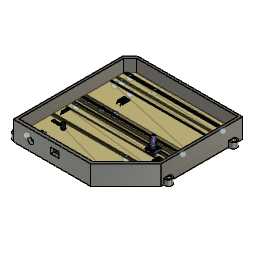
ECE198 Housing v1-4 (Autodesk Fusion 360 design; units mm, degrees)
Autodesk Fusion 360 part; units mm, degrees
note: some values were not read from the file. Set by a fixed rule: which sketch regions a step uses.
other "Base Mesh Feature1"
sketch "Sketch1" plane through (0, 0, 0) normal (0, 0, 1) x (1, 0, 0)
  line L0 (25, 15) -> (591.489777, 15)
  line L1 (401.489777, -615.270017) -> (-15, -615.270017)
  line L2 (591.489777, -425.270017) -> (401.489777, -615.270017)
  line L3 (25, 15) -> (-15, -25)
  line L4 (-15, -615.270017) -> (-15, -25)
  line L5 (-504.56746, -488.736197) -> (-504.56746, -504.009761)
  line L6 (-504.56746, -504.009761) -> (-694.56746, -694.009761)
  arc A0 (-1111.057237, -103.739744) -> (-1111.057237, -138.733703) centre (-1118.560257, -121.236724) ccw
  line L7 (-504.56746, -63.739744) -> (-504.56746, -103.73725)
  line L8 (-1071.057237, -63.739744) -> (-1111.057237, -103.739744)
  line L9 (-1111.057237, -653.739744) -> (-1111.057237, -688.733703)
  arc A1 (-504.573277, -138.733703) -> (-504.56746, -103.73725) centre (-497.070257, -121.236724) ccw
  line L10 (-504.56746, -453.73725) -> (-504.573277, -488.733703)
  arc A2 (-504.573277, -488.733703) -> (-504.56746, -453.73725) centre (-497.070257, -471.236724) ccw
  line L11 (-504.56746, -138.736197) -> (-504.56746, -453.73725)
  line L12 (-504.56746, -103.73725) -> (-504.56746, -138.736197)
  line L13 (-1111.057237, -653.739744) -> (-1111.057237, -138.733703)
  line L14 (-694.56746, -694.009761) -> (-1111.057237, -694.009761)
  arc A3 (-1111.057237, -653.739744) -> (-1111.057237, -688.733703) centre (-1118.560257, -671.236724) ccw
  line L15 (-1071.057237, -63.739744) -> (-504.56746, -63.739744)
  line L16 (-1111.057237, -138.733703) -> (-1111.057237, -103.739744)
  line L17 (-1111.057237, -694.009761) -> (-1111.057237, -688.733703)
  line L18 (591.489777, 15) -> (591.489777, -425.270017)
  point P0 (-15, 15)
  point P1 (591.489777, -615.270017)
  point P2 (-1111.057237, -63.739744)
  point P3 (-504.56746, -694.009761)
  point P4 (-1096.057237, -78.739744)
  dimension "d1" = 190
  dimension "d2" = 190
  dimension "d3" = 40
  dimension "d4" = 40
  dimension "d13" = 190
  dimension "d14" = 190
  dimension "d15" = 40
  dimension "d16" = 40
  constraint horizontal L0
  constraint horizontal L1
  constraint coincident P0 L0
  constraint horizontal L15
  constraint vertical L7
  constraint horizontal L14
  constraint vertical L17
  constraint collinear L13 L17
  constraint collinear L7 L11
  constraint collinear L5 L11
  constraint parallel L13 L16
  constraint perpendicular L0 L18
  measures "d3" distance of P0 L0.start
  measures "d4" distance of P0 L3.end
extrude "Extrude1" add sketch "Sketch1" against normal blind 30 contours L0 L1 L2 L3 L4 L18 picked at (402.659851, -131.756672) makes body 1
sketch "Sketch2" plane through (0, 0, 0) normal (0, 0, 1) x (-1, 0, 0)
  line L0 (-591.489777, -15) -> (-25, -15)
  line L1 (-25, -15) -> (15, 25)
  line L2 (15, 25) -> (15, 615.270017)
  line L3 (15, 615.270017) -> (-401.489777, 615.270017)
  line L4 (-401.489777, 615.270017) -> (-591.489777, 425.270017)
  line L5 (2.339606, 598.31935) -> (-396.106329, 598.31935)
  line L6 (-577.437124, 416.988555) -> (-577.437124, -2.457393)
  line L7 (-577.437124, -2.457393) -> (-32.660394, -2.457393)
  line L8 (2.339606, 32.542607) -> (2.339606, 598.31935)
  line L9 (-32.660394, -2.457393) -> (2.339606, 32.542607)
  line L10 (-577.437124, 416.988555) -> (-396.106329, 598.31935)
  line L11 (-591.489777, 425.270017) -> (-591.489777, -15)
  point P0 (-577.437124, 598.31935)
  point P1 (2.339606, -2.457393)
  dimension "d7" = 35
  dimension "d8" = 35
  constraint horizontal L5
  constraint vertical L6
  constraint horizontal L7
  constraint vertical L8
extrude "Extrude2" add sketch "Sketch2" along normal blind 75 bodies 1
sketch "Sketch3" plane through (0, -615.270017, 0) normal (0, -1, 0) x (1, 0, 0)
  line L0 (-15, 75) -> (-15, -30)
  line L1 (-15, -30) -> (401.489777, -30)
  line L2 (401.489777, -30) -> (401.489777, 75)
  line L3 (401.489777, 75) -> (-15, 75)
  circle A0 centre (78.000001, 20) radius 15.397483
  line L4 (186.579444, 46.059598) -> (230, 46.059598)
  line L5 (230, 46.059598) -> (230, 15)
  line L6 (230, 15) -> (186.579444, 15)
  line L7 (186.579444, 15) -> (186.579444, 46.059598)
  constraint horizontal L4
  constraint vertical L5
  constraint horizontal L6
  constraint vertical L7
extrude "Extrude3" cut sketch "Sketch3" against normal up to surface (16.950668 mm away) contours A0 | L4 L5 L6 L7 picked at (83.132496, 24.453812) picked at (201.052963, 35.706399) bodies 1
sketch "Sketch4" plane through (0, 0, 0) normal (0, 0, 1) x (1, 0, 0)
  line L0 (591.491344, -374.998011) -> (591.485527, -409.994464)
  line L1 (-14.998433, -59.994464) -> (-14.998433, -25.000504)
  arc A0 (591.485527, -59.994464) -> (591.491344, -24.998011) centre (598.988547, -42.497484) ccw
  arc A1 (-14.998433, -575.000504) -> (-14.998433, -609.994464) centre (-22.501453, -592.497484) ccw
  line L2 (591.491344, -24.998011) -> (591.491344, -59.996957)
  arc A2 (591.485527, -409.994464) -> (591.491344, -374.998011) centre (598.988547, -392.497484) ccw
  line L3 (-14.998433, -575.000504) -> (-14.998433, -609.994464)
  line L4 (-14.998433, -615.270521) -> (-14.998433, -609.994464)
  arc A3 (-14.998433, -25.000504) -> (-14.998433, -59.994464) centre (-22.501453, -42.497484) ccw
  point P0 (-14.998433, 14.999496)
  point P1 (0.001567, -0.000504)
  point P2 (591.491344, -615.270521)
  constraint vertical L4
extrude "Extrude4" add sketch "Sketch4" against normal blind 30 bodies 1 makes body 2 at (592.353537, -60.341706, -10)
hole "Hole1" at (603.204735, -392.497609, 0) direction (0, 0, -1) diameter 20 depth 30 tip angle 118 bodies 1
hole "Hole2" at (-26.716241, -592.497484, 0) direction (0, 0, -1) diameter 20 depth 30 tip angle 118 bodies 1
hole "Hole3" at (-26.716241, -42.497484, 0) direction (0, 0, -1) diameter 20 depth 30 tip angle 118 bodies 1
hole "Hole4" at (603.205392, -42.497484, 0) direction (0, 0, -1) diameter 22 depth 30 tip angle 118 bodies 2
sketch "Sketch5" plane through (0, 0, 0) normal (0, 0, 1) x (-1, 0, 0)
  line L0 (-32.660394, -2.457393) -> (2.339606, 32.542607)
  line L1 (2.339606, 32.542607) -> (2.339606, 598.31935)
  line L2 (2.339606, 598.31935) -> (-396.106329, 598.31935)
  line L3 (-396.106329, 598.31935) -> (-577.437124, 416.988555)
  line L4 (-577.437124, 416.988555) -> (-577.437124, -2.457393)
  line L5 (-577.437124, -2.457393) -> (-32.660394, -2.457393)
  circle A0 centre (-164.601236, 245.898781) radius 7.211103
  circle A1 centre (-20.502491, 309.415277) radius 7.211103
  circle A2 centre (-399.476491, 420.58754) radius 7.211103
  circle A3 centre (-20.683938, 579.474554) radius 7.211103
  circle A4 centre (-164.813294, 29.373002) radius 7.211103
  circle A5 centre (-30.212747, 29.594938) radius 7.211103
  circle A6 centre (-530.651177, 29.416112) radius 7.211103
  circle A7 centre (-164.601236, 245.898781) radius 7.211103
  circle A8 centre (-530.657462, 245.579878) radius 7.211103
  circle A9 centre (-164.601236, 245.898781) radius 7.211103
  circle A10 centre (-399.722447, 280.089299) radius 7.211103
  circle A11 centre (-164.601236, 245.898781) radius 7.211103
  circle A12 centre (-105.000002, 259.500004) radius 3.941266
  circle A13 centre (-105.000002, 259.500004) radius 3.941266
  circle A14 centre (-25.000002, 259.500004) radius 3.941266
  circle A15 centre (-105.000002, 106.000004) radius 3.941266
  circle A16 centre (-25.000002, 106.000004) radius 3.941266
  circle A17 centre (-31.590682, 73.221195) radius 5.64287
  point P0 (-105.000002, 259.500004)
equation "d2 = d1"
equation "d4 = d3"
equation "d8 = d7"
equation "d14 = d1"
equation "d16 = d3"
